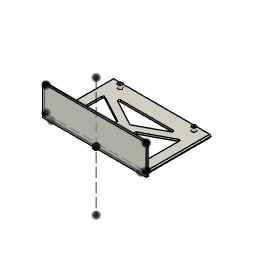
Mainboard Mount Pro - BLANK (Autodesk Fusion 360 design; units mm, degrees)
Autodesk Fusion 360 part; units mm, degrees
sketch "Sketch13" plane through (0, 0, 0) normal (0, 0, -1) x (1, 0, 0)
  line L0 (0.9482, -57.3251) -> (45.3598, -81.2391)
  arc A0 (44.4116, -85) -> (45.3598, -81.2391) centre (44.4116, -83) ccw
  line L1 (44.4116, -85) -> (-44.4116, -85)
  arc A1 (-45.3598, -81.2391) -> (-44.4116, -85) centre (-44.4116, -83) ccw
  line L2 (-45.3598, -81.2391) -> (-0.9482, -57.3251)
  arc A2 (0.9482, -57.3251) -> (-0.9482, -57.3251) centre (0, -59.086) ccw
  line L3 (65, -25.163) -> (65, -74.837)
  arc A3 (62.0518, -76.598) -> (65, -74.837) centre (63, -74.837) ccw
  line L4 (62.0518, -76.598) -> (15.9259, -51.7609)
  arc A4 (15.9259, -48.2391) -> (15.9259, -51.7609) centre (16.8741, -50) ccw
  line L5 (15.9259, -48.2391) -> (62.0518, -23.402)
  arc A5 (65, -25.163) -> (62.0518, -23.402) centre (63, -25.163) ccw
  line L6 (-62.0518, -23.402) -> (-15.9259, -48.2391)
  arc A6 (-15.9259, -51.7609) -> (-15.9259, -48.2391) centre (-16.8741, -50) ccw
  line L7 (-15.9259, -51.7609) -> (-62.0518, -76.598)
  arc A7 (-65, -74.837) -> (-62.0518, -76.598) centre (-63, -74.837) ccw
  line L8 (-65, -74.837) -> (-65, -25.163)
  arc A8 (-62.0518, -23.402) -> (-65, -25.163) centre (-63, -25.163) ccw
  line L9 (45.3598, -18.7609) -> (0.9482, -42.6749)
  arc A9 (-0.9482, -42.6749) -> (0.9482, -42.6749) centre (0, -40.914) ccw
  line L10 (-0.9482, -42.6749) -> (-45.3598, -18.7609)
  arc A10 (-44.4116, -15) -> (-45.3598, -18.7609) centre (-44.4116, -17) ccw
  line L11 (-44.4116, -15) -> (44.4116, -15)
  arc A11 (45.3598, -18.7609) -> (44.4116, -15) centre (44.4116, -17) ccw
  line L12 (82.8, 0) -> (87, 0)
  line L13 (87, 0) -> (87, 3)
  line L14 (87, 3) -> (-87, 3)
  line L15 (-87, 3) -> (-87, 0)
  line L16 (-87, 0) -> (-82.8, 0)
  line L17 (-82.8, 0) -> (-82.8, -110)
  line L18 (-82.8, -110) -> (82.8, -110)
  line L19 (82.8, -110) -> (82.8, 0)
  line L20 (65.8, -110) -> (50.8, -110)
  line L21 (50.8, -110) -> (50.8, -60)
  line L22 (50.8, -60) -> (65.8, -60)
  line L23 (65.8, -60) -> (65.8, -110)
  line L24 (-38.8, -110) -> (-53.8, -110)
  line L25 (-53.8, -110) -> (-53.8, -2)
  line L26 (-53.8, -2) -> (-38.8, -2)
  line L27 (-38.8, -2) -> (-38.8, -110)
  dimension "d1" = 15
  dimension "d2" = 15
  dimension "d3" = 17
  dimension "d4" = 50
  dimension "d5" = 108
  dimension "d6" = 29
  constraint horizontal L20
  constraint vertical L21
  constraint horizontal L22
  constraint vertical L23
  constraint coincident L18 L20.start
  constraint horizontal L24
  constraint vertical L25
  constraint horizontal L26
  constraint vertical L27
  measures "d1" distance of L21 L23
  measures "d2" distance of L25 L27
  measures "d3" distance of L19 L23
  measures "d4" distance of L20.start L22.end
  measures "d5" distance of L24.end L25.end
  measures "d6" distance of L17 L25
sketch "Sketch14" plane through (0, 0, 0) normal (0, 0, -1) x (1, 0, 0)
  line L0 (-62.0518, -23.402) -> (-15.9259, -48.2391)
  arc A0 (-15.9259, -51.7609) -> (-15.9259, -48.2391) centre (-16.8741, -50) ccw
  line L1 (-15.9259, -51.7609) -> (-62.0518, -76.598)
  arc A1 (-65, -74.837) -> (-62.0518, -76.598) centre (-63, -74.837) ccw
  line L2 (-65, -74.837) -> (-65, -25.163)
  arc A2 (-62.0518, -23.402) -> (-65, -25.163) centre (-63, -25.163) ccw
  line L3 (-0.9482, -42.6749) -> (-45.3598, -18.7609)
  arc A3 (-44.4116, -15) -> (-45.3598, -18.7609) centre (-44.4116, -17) ccw
  line L4 (-44.4116, -15) -> (44.4116, -15)
  arc A4 (45.3598, -18.7609) -> (44.4116, -15) centre (44.4116, -17) ccw
  line L5 (45.3598, -18.7609) -> (0.9482, -42.6749)
  arc A5 (-0.9482, -42.6749) -> (0.9482, -42.6749) centre (0, -40.914) ccw
  line L6 (-82.8, -110) -> (82.8, -110)
  line L7 (82.8, -110) -> (82.8, 0)
  line L8 (82.8, 0) -> (87, 0)
  line L9 (87, 0) -> (87, 3)
  line L10 (87, 3) -> (-87, 3)
  line L11 (-87, 3) -> (-87, 0)
  line L12 (-87, 0) -> (-82.8, 0)
  line L13 (-82.8, 0) -> (-82.8, -110)
  line L14 (44.4116, -85) -> (-44.4116, -85)
  arc A6 (-45.3598, -81.2391) -> (-44.4116, -85) centre (-44.4116, -83) ccw
  line L15 (-45.3598, -81.2391) -> (-0.9482, -57.3251)
  arc A7 (0.9482, -57.3251) -> (-0.9482, -57.3251) centre (0, -59.086) ccw
  line L16 (0.9482, -57.3251) -> (45.3598, -81.2391)
  arc A8 (44.4116, -85) -> (45.3598, -81.2391) centre (44.4116, -83) ccw
  line L17 (62.0518, -76.598) -> (15.9259, -51.7609)
  arc A9 (15.9259, -48.2391) -> (15.9259, -51.7609) centre (16.8741, -50) ccw
  line L18 (15.9259, -48.2391) -> (62.0518, -23.402)
  arc A10 (65, -25.163) -> (62.0518, -23.402) centre (63, -25.163) ccw
  line L19 (65, -25.163) -> (65, -74.837)
  arc A11 (62.0518, -76.598) -> (65, -74.837) centre (63, -74.837) ccw
  line L20 (65.3, -110) -> (51.3, -110)
  line L21 (51.3, -110) -> (51.3, -61)
  line L22 (51.3, -61) -> (65.3, -61)
  line L23 (65.3, -61) -> (65.3, -110)
  line L24 (-39.3, -110) -> (-53.3, -110)
  line L25 (-53.3, -110) -> (-53.3, -3)
  line L26 (-53.3, -3) -> (-39.3, -3)
  line L27 (-39.3, -3) -> (-39.3, -110)
  dimension "d7" = 107
  dimension "d8" = 49
  dimension "d9" = 14
  dimension "d10" = 14
  dimension "d11" = 29.5
  dimension "d12" = 17.5
  constraint horizontal L20
  constraint vertical L21
  constraint horizontal L22
  constraint vertical L23
  constraint coincident L6 L20.start
  constraint horizontal L24
  constraint vertical L25
  constraint horizontal L26
  constraint vertical L27
  constraint coincident L6 L24.start
  measures "d7" distance of L24.end L25.end
  measures "d8" distance of L20.start L22.end
  measures "d9" distance of L21 L23
  measures "d10" distance of L25 L27
  measures "d11" distance of L13 L25
  measures "d12" distance of L7 L23
sketch "Sketch1" plane through (0, 0, 0) normal (0, 1, 0) x (1, 0, 0)
  line L0 (-75, 0) -> (75, 0) construction
  line L1 (-87, -50) -> (87, -50)
  line L2 (87, -50) -> (87, 0)
  line L3 (87, 0) -> (-87, 0)
  line L4 (-87, 0) -> (-87, -50)
  line L5 (0, -100) -> (0, 100) construction
  circle A0 centre (-84, -47) radius 1.75
  circle A1 centre (-84, -47) radius 3
  circle A2 centre (-84, -6.75) radius 1.75
  circle A3 centre (-84, -6.75) radius 3
  circle A4 centre (84, -47) radius 1.75
  circle A5 centre (84, -47) radius 3
  circle A6 centre (84, -6.75) radius 1.75
  circle A7 centre (84, -6.75) radius 3
  line L6 (-87, -5) -> (87, -5) construction
  dimension "d99_1" = 150
  dimension "d100_1" = 174
  dimension "d101_1" = 50
  dimension "d102_1" = 200
  dimension "d103_1" = 3.5
  dimension "d104_1" = 6
  dimension "d105_1" = 3.5
  dimension "d106_1" = 6
  dimension "d107_1" = 3.5
  dimension "d108_1" = 6
  dimension "d109_1" = 3.5
  dimension "d110_1" = 6
  dimension "d111_1" = 5
  constraint horizontal L0
  constraint midpoint L0 origin
  constraint horizontal L1
  constraint vertical L2
  constraint horizontal L3
  constraint vertical L4
  constraint vertical L5
  constraint midpoint L5 origin
  constraint midpoint L3 origin
  constraint coincident L5 origin
  constraint concentric A0 A1
  constraint concentric A2 A3
  constraint concentric A4 A5
  constraint concentric A6 A7
  constraint horizontal A0.centre A4.centre
  constraint vertical A4.centre A6.centre
  constraint vertical A0.centre A2.centre
  constraint horizontal A2.centre A6.centre
  constraint tangent L1 A1
  constraint tangent L4 A1
  constraint tangent L2 A5
  constraint coincident L4 L6.start
  constraint coincident L2 L6.end
  constraint perpendicular L2 L6
  constraint tangent A6 L6
  measures "d99_1" distance of L0.start L0.end
  measures "d100_1" distance of L1.start L1.end
  measures "d101_1" distance of L1.start L3.end
  measures "d102_1" distance of L5.start L5.end
  measures "d103_1" diameter of A0
  measures "d104_1" diameter of A1
  measures "d105_1" diameter of A2
  measures "d106_1" diameter of A3
  measures "d107_1" diameter of A4
  measures "d108_1" diameter of A5
  measures "d109_1" diameter of A6
  measures "d110_1" diameter of A7
  measures "d111_1" distance of L3 L6
extrude "Extrude1" add sketch "Sketch1" against normal blind 3 contours L1 L4 A1 | A7 | A3 | L1 L2 L3 L4 A1 A5 | A1 | L1 L2 A5 | A5
sketch "Sketch2" plane through (0, 0, 0) normal (0, 1, 0) x (-1, 0, 0)
  circle A0 centre (-84, 6.75) radius 1.75
  circle A1 centre (-84, 47) radius 1.75
  circle A2 centre (84, 6.75) radius 1.75
  circle A3 centre (84, 47) radius 1.75
  line L0 (87, 50) -> (-87, 50)
  line L1 (-87, 50) -> (-87, 0)
  line L2 (-87, 0) -> (87, 0)
  line L3 (87, 0) -> (87, 50)
  line L4 (-87, 3) -> (87, 3)
  line L5 (-82.8, 0) -> (-82.8, 1)
  line L6 (-82.8, 1) -> (-80.8, 3)
  line L7 (-82.8, 1) -> (82.8, 1) construction
  line L8 (82.8, 0) -> (82.8, 1)
  line L9 (82.8, 1) -> (80.8, 3)
  line L10 (0, 70.9993) -> (0, -26.0281) construction
  line L11 (0, 100) -> (0, -100)
  point P0 (0, 1)
  dimension "d114_1" = 3
  dimension "d115_1" = 1
  dimension "d116_1" = 45
  dimension "d118_1" = 1
  dimension "d119_1" = 135
  dimension "d18" = 165.6
  constraint coincident L1 L4.start
  constraint coincident L3 L4.end
  constraint perpendicular L3 L4
  constraint coincident L2 L5.start
  constraint perpendicular L2 L5
  constraint horizontal L7
  constraint coincident L4 L6.end
  constraint perpendicular L2 L8
  constraint coincident L4 L9.end
  constraint coincident L2 L8.start
  constraint midpoint L7 P0
  constraint perpendicular L4 L10
  constraint coincident L10 origin
  constraint coincident P0 L11
  measures "d114_1" distance of L2 L4
  measures "d115_1" distance of L5.start L5.end
  measures "d116_1" angle of L6 L7
  measures "d118_1" distance of L8.start L7.end
  measures "d119_1" angle of L8 L9
  measures "d18" distance of L5 L8
extrude "Extrude22" add sketch "Sketch2" along normal blind 8 contours L2 L4 L5 L6 L11 | L2 L4 L8 L9 L11
extrude "Extrude2" add sketch "Sketch2" along normal blind 110 contours L2 L4 L5 L6 L11 | L2 L4 L8 L9 L11
sketch "Sketch3" plane through (0, 0, 3) normal (0, 0, 1) x (-1, 0, 0)
  line L0 (80.8, 0) -> (-80.8, 0)
  line L1 (-80.8, 0) -> (-80.8, -110)
  line L2 (-80.8, -110) -> (80.8, -110)
  line L3 (80.8, -110) -> (80.8, 0)
  line L4 (0, 0) -> (0, -110) construction
  line L5 (82.8, 0, -3) -> (82.8, -110, -3) construction
  line L6 (82.8, -55, -3) -> (62.187, -54.4724, -3.177) construction
  line L7 (-82.8, 0, -2) -> (-82.8, -110, -2) construction
  line L8 (62.187, -54.4724, -3.177) -> (-82.8, -55, -2) construction
  circle A0 centre (62, -15.75) radius 1.45
  circle A1 centre (62, -15.75) radius 3.5
  circle A2 centre (62, -102.25) radius 1.45
  circle A3 centre (62, -102.25) radius 3.5
  circle A4 centre (-62, -15.75) radius 1.45
  circle A5 centre (-62, -15.75) radius 3.5
  circle A6 centre (-62, -102.25) radius 1.45
  circle A7 centre (-62, -102.25) radius 3.5
  line L9 (65, -85) -> (-65, -85)
  line L10 (-65, -85) -> (-65, -15)
  line L11 (-65, -15) -> (65, -15)
  line L12 (65, -15) -> (65, -85)
  line L13 (65, -15) -> (-65, -85) construction
  line L14 (65, -85) -> (-65, -15) construction
  line L15 (65, -78.1855) -> (12.6556, -50)
  line L16 (0, -43.1855) -> (-52.3444, -15)
  line L17 (52.3444, -85) -> (0, -56.8145)
  line L18 (-12.6556, -50) -> (-65, -21.8145)
  line L19 (65, -21.8145) -> (12.6556, -50)
  line L20 (0, -56.8145) -> (-52.3444, -85)
  line L21 (52.3444, -15) -> (0, -43.1855)
  line L22 (-12.6556, -50) -> (-65, -78.1855)
  line L23 (73.5, 0) -> (-73.5, 0) construction
  line L24 (-73.5, 0) -> (-73.5, -95) construction
  line L25 (-73.5, -95) -> (73.5, -95) construction
  line L26 (73.5, -95) -> (73.5, 0) construction
  point P0 (0, -55)
  dimension "d124_1" = 2.9
  dimension "d125_1" = 7
  dimension "d126_1" = 2.9
  dimension "d127_1" = 7
  dimension "d128_1" = 2.9
  dimension "d129_1" = 7
  dimension "d130_1" = 2.9
  dimension "d131_1" = 7
  dimension "d132_1" = 86.5
  dimension "d133_1" = 124
  dimension "d134_1" = 15.75
  dimension "d149_1" = 130
  dimension "d150_1" = 70
  dimension "d154_1" = 6
  dimension "d31" = 147
  dimension "d32" = 95
  dimension "d33" = 6
  dimension "d34" = 15
  dimension "d35" = 6
  dimension "d175" = 86.5
  constraint coincident L4.start origin
  constraint midpoint L2 L4.end
  constraint concentric A0 A1
  constraint concentric A2 A3
  constraint concentric A4 A5
  constraint concentric A6 A7
  constraint vertical A0.centre A2.centre
  constraint horizontal A0.centre A4.centre
  constraint horizontal A2.centre A6.centre
  constraint vertical A4.centre A6.centre
  constraint symmetric L4 A2.centre A6.centre
  constraint horizontal L9
  constraint vertical L10
  constraint horizontal L11
  constraint vertical L12
  constraint symmetric L4 L10 L12
  constraint midpoint L4 P0
  constraint coincident L9 L17.start
  constraint coincident L10 L18.end
  constraint coincident L12 L15.start
  constraint coincident L11 L16.end
  constraint parallel L15 L17
  constraint coincident L12 L19.start
  constraint coincident L9 L20.end
  constraint coincident L11 L21.start
  constraint coincident L10 L22.end
  constraint parallel L19 L21
  constraint parallel L13 L21
  constraint parallel L14 L17
  constraint coincident L4 L16.start
  constraint coincident L4 L17.end
  constraint coincident L18.start L21
  constraint collinear L19 L20
  constraint collinear L21 L22
  constraint vertical L24
  constraint horizontal L25
  constraint vertical L26
  constraint coincident L0 L23.start
  constraint symmetric L4 L24 L26
  constraint collinear L15 L16
  measures "d124_1" diameter of A0
  measures "d125_1" diameter of A1
  measures "d126_1" diameter of A2
  measures "d127_1" diameter of A3
  measures "d128_1" diameter of A4
  measures "d129_1" diameter of A5
  measures "d130_1" diameter of A6
  measures "d131_1" diameter of A7
  measures "d132_1" distance of A0.centre A2.centre
  measures "d133_1" distance of A2.centre A6.centre
  measures "d134_1" distance of L0 A0.centre
  measures "d149_1" distance of L9.start L9.end
  measures "d150_1" distance of L9 L11
  measures "d154_1" distance of L13 L21
  measures "d31" distance of L24.end L25.end
  measures "d32" distance of L23 L25
  measures "d33" distance of L14 L18
  measures "d34" distance of L11 L23.start
  measures "d35" distance of L14 L15
  measures "d175" distance of A0.centre A2.centre
extrude "Extrude6" cut sketch "Sketch3" against normal blind 3 contours L11 L16 L21 | L12 L15 L19 | L9 L17 L20 | L10 L18 L22
extrude "Extrude3" add sketch "Sketch3" along normal blind 6 contours A0 A1 L11 L12 | A0 A1 L11 L12 | A4 A5 L10 L11 | A4 A5 L10 L11 | A3 | A7
fillet "Fillet1" radius 2 12 edges at (-52.3444, 85, 1.5) (12.6556, 50, 1.5) (0, 56.8145, 1.5) (-12.6556, 50, 1.5) (0, 43.1855, 1.5) (52.3444, 85, 1.5) (-65, 21.8145, 1.5) (-65, 78.1855, 1.5) (65, 78.1855, 1.5) (65, 21.8145, 1.5) (52.3444, 15, 1.5) (-52.3444, 15, 1.5)
extrude "Extrude31" [suppressed]
chamfer "Chamfer38" [suppressed]
chamfer "Chamfer39" [suppressed]
chamfer "Chamfer40" [suppressed]
chamfer "Chamfer41" [suppressed]
chamfer "Chamfer42" [suppressed]
extrude "Extrude32" [suppressed]
chamfer "Chamfer43" [suppressed]
